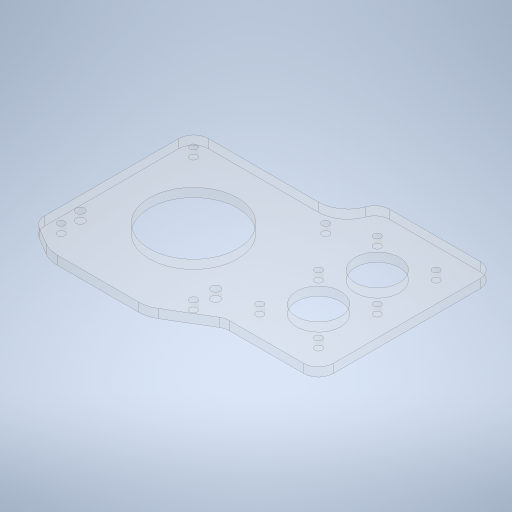
# Autodesk Inventor part: TransmissionDeck
Saved by Autodesk Inventor 2023 (Build 270158000, 158)
## iProperties
Created: 2022-11-08
Part Number: TransmissionDeck
Material: Polycarbonate, Clear
Document SubType Name: Modeling
Designer: Administrator
Density: 1.2 g/cm^3
Appearance: Polycarbonate - Clear
Author: Administrator
Autodesk Inventor part; units mm, degrees
ref_plane "YZ Plane" through (0, 0, 0) normal (1, 0, 0) x (0, 1, 0)
ref_plane "XZ Plane" through (0, 0, 0) normal (0, 1, 0) x (-1, 0, 0)
ref_plane "XY Plane" through (0, 0, 0) normal (0, 0, 1) x (1, 0, 0)
sketch "Sketch1" plane through (0, 0, 0) normal (0, 1, 0) x (-1, 0, 0)
  line L0 (10, 0) -> (80, 0)
  line L1 (90, -32.6619) -> (90, -167.3381)
  line L2 (67, -200) -> (23, -200)
  line L3 (0, -167.3381) -> (0, -85)
  line L4 (68, -27) -> (68, -173) construction
  line L5 (68, -173) -> (22, -173) construction
  line L6 (22, -173) -> (22, -27) construction
  circle A0 centre (68, -27) radius 1.5
  circle A1 centre (68, -173) radius 1.5
  circle A2 centre (22, -173) radius 1.5
  circle A3 centre (22, -27) radius 1.5
  line L7 (30, -70) -> (60, -70)
  line L8 (70, -80) -> (70, -120)
  line L9 (60, -130) -> (30, -130)
  line L10 (20, -120) -> (20, -80)
  arc A4 (70, -80) -> (60, -70) centre (60, -80) ccw
  arc A5 (60, -130) -> (70, -120) centre (60, -120) ccw
  arc A6 (20, -120) -> (30, -130) centre (30, -120) ccw
  arc A7 (30, -70) -> (20.5719, -76.6667) centre (30, -80) ccw
  arc A8 (90, -10) -> (80, 0) centre (80, -10) ccw
  arc A9 (0, -190) -> (10, -200) centre (10, -190) ccw
  arc A10 (80, -200) -> (90, -190) centre (80, -190) ccw
  arc A11 (10, 0) -> (0, -10) centre (10, -10) ccw
  circle A12 centre (80, -10) radius 1.25
  circle A13 centre (80, -30) radius 1.25
  circle A14 centre (80, -50) radius 1.25
  circle A15 centre (80, -70) radius 1.25
  circle A16 centre (80, -90) radius 1.25
  circle A17 centre (80, -110) radius 1.25
  circle A18 centre (80, -130) radius 1.25
  circle A19 centre (80, -150) radius 1.25
  circle A20 centre (80, -170) radius 1.25
  circle A21 centre (80, -190) radius 1.25
  circle A22 centre (10, -10) radius 1.25
  circle A23 centre (10, -30) radius 1.25
  circle A24 centre (10, -50) radius 1.25
  circle A25 centre (10, -70) radius 1.25
  circle A26 centre (10, -90) radius 1.25
  circle A27 centre (10, -110) radius 1.25
  circle A28 centre (10, -130) radius 1.25
  circle A29 centre (10, -150) radius 1.25
  circle A30 centre (10, -170) radius 1.25
  circle A31 centre (10, -190) radius 1.25
  circle A32 centre (81, -111) radius 3.5
  circle A33 centre (81.25, -89) radius 3.5
  circle A34 centre (9, -111) radius 3.5
  circle A35 centre (9, -89) radius 3.5
  line L11 (70.0725, -15.0435) -> (64.0418, -11.4251)
  line L12 (12.8542, -19.2875) -> (25.9582, -11.4251)
  arc A36 (90, -32.6619) -> (85.145, -24.087) centre (80, -32.6619) ccw
  arc A37 (4.855, -24.087) -> (0, -32.6619) centre (10, -32.6619) ccw construction
  circle A38 centre (67.5, -65) radius 1.25
  circle A39 centre (22.5, -65) radius 1.25
  line L13 (-15, -70) -> (15, -70)
  circle A40 centre (67.5, -20) radius 1.25
  line L14 (30, -25) -> (60, -25)
  circle A41 centre (22.5, -20) radius 1.25
  line L15 (-15, -25) -> (15, -25) construction
  line L16 (58.8968, -10) -> (31.1032, -10)
  arc A42 (64.0418, -11.4251) -> (58.8968, -10) centre (58.8968, -20) ccw
  arc A43 (31.1032, -10) -> (25.9582, -11.4251) centre (31.1032, -20) ccw
  line L17 (90, -200) -> (72, -200) construction
  line L18 (72, -195) -> (72, -185)
  line L19 (77, -180) -> (85, -180)
  line L20 (90, -175) -> (90, -167.3381)
  line L21 (0, -200) -> (18, -200) construction
  line L22 (18, -195) -> (18, -185)
  line L23 (13, -180) -> (5, -180)
  line L24 (0, -175) -> (0, -167.3381)
  arc A44 (77, -180) -> (72, -185) centre (77, -185) ccw
  arc A45 (85, -180) -> (90, -175) centre (85, -175) ccw
  arc A46 (0, -175) -> (5, -180) centre (5, -175) ccw
  arc A47 (18, -185) -> (13, -180) centre (13, -185) ccw
  arc A48 (67, -200) -> (72, -195) centre (67, -195) ccw
  arc A49 (18, -195) -> (23, -200) centre (23, -195) ccw
  circle A50 centre (69.1385, -144.2) radius 1.25
  circle A51 centre (20.8615, -144.2) radius 1.25
  circle A52 centre (53.8985, -195) radius 1.25
  line L25 (10, -30) -> (-10, -30) construction
  line L26 (-10, -30) -> (-10, -50) construction
  line L27 (-10, -50) -> (10, -50) construction
  line L28 (10, -50) -> (10, -30) construction
  circle A53 centre (-10, -50) radius 1.25
  circle A54 centre (-10, -30) radius 1.25
  line L29 (-10, -30) -> (-10, -20) construction
  line L30 (-10, -20) -> (10.2817, -20)
  line L31 (-10, -20) -> (-15, -20)
  line L32 (-20, -25) -> (-20, -75)
  line L33 (-15, -80) -> (-5, -80)
  arc A55 (-15, -20) -> (-20, -25) centre (-15, -25) ccw
  arc A56 (-20, -75) -> (-15, -80) centre (-15, -75) ccw
  arc A57 (0, -85) -> (-5, -80) centre (-5, -85) ccw
  arc A58 (10.2817, -20) -> (12.8542, -19.2875) centre (10.2817, -15) ccw
  line L34 (-10, -50) -> (-10, -70) construction
  circle A59 centre (-10, -70) radius 1.25
  line L35 (-10, -80) -> (15.8579, -80)
  line L36 (60, -70) -> (67.5, -70)
  line L37 (72.5, -65) -> (72.5, -19.331)
  arc A60 (72.5, -19.331) -> (70.0725, -15.0435) centre (67.5, -19.331) ccw
  arc A61 (67.5, -70) -> (72.5, -65) centre (67.5, -65) ccw
  arc A62 (15.8579, -80) -> (20.5719, -76.6667) centre (15.8579, -75) ccw
  line L38 (10, -70) -> (-10, -50) construction
  line L39 (10, -30) -> (-10, -50) construction
  circle A63 centre (0, -60) radius 7.5
  circle A64 centre (0, -40) radius 7.5
  line L40 (67.5, -65) -> (22.5, -20) construction
  circle A65 centre (45, -42.5) radius 15
  point P0 (0, 0)
  point P1 (90, 0)
  point P2 (70, -130)
  point P3 (70, -70)
  point P4 (20, -130)
  point P5 (45, 0)
  point P6 (45, -200)
  point P7 (25, -70)
  point P8 (70, -25)
  point P9 (25, -25)
  point P10 (72, -180)
  point P11 (-20, -20)
  point P12 (-20, -80)
  point P13 (72.5, -70)
  dimension "d0" = 90
  dimension "d1" = 200
  dimension "d2" = 46
  dimension "d4" = 22
  dimension "d5" = 27
  dimension "d7" = 3
  dimension "d8" = 3
  dimension "d10" = 50
  dimension "d11" = 60
  dimension "d12" = 20
  dimension "d13" = 70
  dimension "d14" = 10
  dimension "d15" = 10
  dimension "d16" = 2.5
  dimension "d19" = 20
  dimension "d24" = 2.5
  dimension "d27" = 20
  dimension "d34" = 7
  dimension "d35" = 7
  dimension "d36" = 7
  dimension "d37" = 7
  dimension "d38" = 72
  dimension "d39" = 22
  dimension "d40" = 9
  dimension "d41" = 89
  dimension "d42" = 22
  dimension "d43" = 72
  dimension "d46" = 10
  dimension "d48" = 2.5
  dimension "d51" = 45
  dimension "d54" = 45
  dimension "d57" = 22.5
  dimension "d58" = 5
  dimension "d71" = 18
  dimension "d72" = 20
  dimension "d73" = 18
  dimension "d74" = 5
  dimension "d75" = 5
  dimension "d76" = 2.5
  dimension "d77" = 2.5
  dimension "d78" = 0
  dimension "d79" = 48.277
  dimension "d81" = 20.8615
  dimension "d82" = 2.5
  dimension "d83" = 15.24
  dimension "d84" = 50.8
  dimension "d85" = 5
  dimension "d86" = 20
  dimension "d87" = 20
  dimension "d88" = 2.5
  dimension "d89" = 2.5
  dimension "d92" = 10
  dimension "d93" = 10
  dimension "d94" = 60
  dimension "d95" = 5
  dimension "d96" = 5
  dimension "d97" = 20
  dimension "d98" = 2.5
  dimension "d99" = 12.5
  dimension "d100" = 5
  dimension "d101" = 5
  dimension "d102" = 15
  dimension "d103" = 15
  dimension "d104" = 30
  constraints: 80 end point, 66 centre point, 51 point on circle, 46 tangent, 35 point on line, 15 equal radius, 12 perpendicular, 9 coincident, 8 horizontal, 6 parallel, 5 midpoint, 5 vertical, 1 collinear, 67 other
  measures "d0" distance of L17.start L21.start
  measures "d1" distance of point (90, 0) L17.start
  measures "d2" distance of L4.end L5.end
  measures "d4" distance between parallel lines of L1 L4
  measures "d7" diameter of A1
  measures "d8" diameter of A2
  measures "d10" distance of point (70, -130) point (20, -130)
  measures "d11" distance of point (70, -70) point (70, -130)
  measures "d12" distance between parallel lines of L3 L10
  measures "d13" distance between parallel lines of L0 L7
  measures "d14" radius of A4
  measures "d15" radius of A8
  measures "d16" diameter of A12
  measures "d19" distance of A12.centre A13.centre
  measures "d24" diameter of A22
  measures "d27" distance of A22.centre L25.start
  measures "d34" diameter of A32
  measures "d35" diameter of A33
  measures "d36" diameter of A34
  measures "d37" diameter of A35
  measures "d38" distance of A34.centre A32.centre
  measures "d39" distance of A35.centre A34.centre
  measures "d40" distance from line of L3 A34.centre
  measures "d42" vertical distance of A34.centre A33.centre
  measures "d43" horizontal distance of A35.centre A32.centre
  measures "d46" radius of A36
  measures "d48" diameter of A38
  measures "d51" distance of A38.centre A39.centre
  measures "d54" distance of A38.centre A40.centre
  measures "d57" distance from line of L1 A38.centre
  measures "d58" distance from line of L7 A38.centre
  measures "d71" distance of L17.start L17.end
  measures "d72" distance of L17.end point (72, -180)
  measures "d73" distance of L21.start L21.end
  measures "d74" radius of A44
  measures "d75" radius of A48
  measures "d76" diameter of A50
  measures "d77" diameter of A51
  measures "d78" vertical distance of A51.centre A50.centre
  measures "d79" distance of A51.centre A50.centre
  measures "d81" distance from line of L3 A51.centre
  measures "d82" diameter of A52
  measures "d83" horizontal distance of A52.centre A50.centre
  measures "d84" vertical distance of A50.centre A52.centre
  measures "d86" distance of L27.end L26.end
  measures "d87" distance of L26.end L25.end
  measures "d88" diameter of A53
  measures "d89" diameter of A54
  measures "d92" distance of L29.start L29.end
  measures "d93" distance of L29.end point (-20, -20)
  measures "d94" distance of point (-20, -20) point (-20, -80)
  measures "d95" radius of A55
  measures "d96" radius of A58
  measures "d97" distance of L34.start L34.end
  measures "d98" diameter of A59
  measures "d99" distance of L7.end point (72.5, -70)
  measures "d100" radius of A60
  measures "d101" radius of A62
  measures "d102" diameter of A63
  measures "d103" diameter of A64
  measures "d104" diameter of A65
extrude "Extrusion2" add sketch "Sketch1" along normal blind 3 contours A7 A62 L35 L33 A56 L32 A55 L31 L30 A58 L12 A43 L16 A42 L11 A60 L37 A61 L36 L7
equation "\"d4\" = -0.5 * d2 + 0.5 * d0"
equation "\"d5\" = -0.5 * d3 + 0.5 * d1"
equation "\"d12\" = -0.5 * d10 + 0.5 * d0"
equation "\"d13\" = -0.5 * d11 + 0.5 * d1"
equation "\"d40\" = -0.5 * d38 + 0.5 * d0"
equation "\"d41\" = -0.5 * d39 + 0.5 * d1"
equation "\"d57\" = -0.5 * d51 + 0.5 * d0"
equation "\"d81\" = -0.5 * d79 + 0.5 * d0"
equation "\"d3\" = 146"
body "Solid2"
